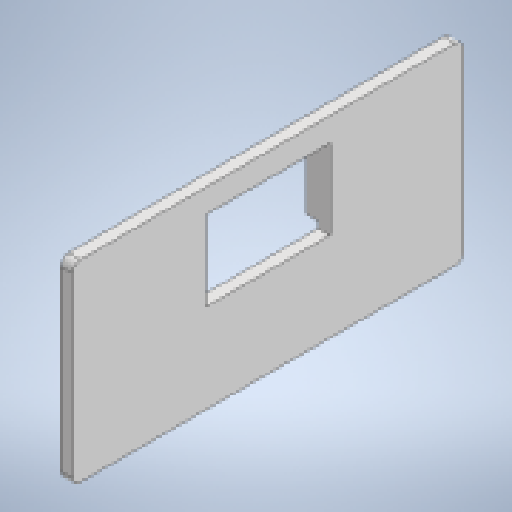
# Autodesk Inventor part: pokrywa_tyl
Saved by Autodesk Inventor 2023 (Build 270158000, 158)
## iProperties
Created: 2024-07-28
Part Number: pokrywa_tyl
Material: Ogólny
Document SubType Name: Modeling
Designer: kamil
Density: 1 g/cm^3
Appearance: Domyślna
Author: kamil
Autodesk Inventor part; units mm, degrees
ref_plane "YZ Plane" through (0, 0, 0) normal (1, 0, 0) x (0, 1, 0)
ref_plane "XZ Plane" through (0, 0, 0) normal (0, 1, 0) x (-1, 0, 0)
ref_plane "XY Plane" through (0, 0, 0) normal (0, 0, 1) x (1, 0, 0)
sketch "Szkic1" plane through (0, 0, 0) normal (1, 0, 0) x (0, 1, 0)
  line L0 (-29.4319, -23.6453) -> (19.8681, -23.6453)
  line L1 (19.8681, -23.6453) -> (19.8681, 76.3547)
  line L2 (19.8681, 76.3547) -> (-29.4319, 76.3547)
  line L3 (-29.4319, 76.3547) -> (-29.4319, -23.6453)
  point P0 (0, 0)
  dimension "d0" = 100
  dimension "d1" = 49.3
  constraints: 8 end point, 2 parallel, 1 horizontal, 1 perpendicular
  measures "d0" distance of L0.end L1.end
  measures "d1" distance between parallel lines of L3 L1
extrude "Wyciągnięcie proste1" add sketch "Szkic1" along normal blind 3
fillet "Zaokrąglenie1" radius 2 4 edges at (1.5, 19.8681, 76.3547) (1.5, -29.4319, 76.3547) (1.5, -29.4319, -23.6453) (1.5, 19.8681, -23.6453)
sketch "Szkic3" plane through (3, 0, 0) normal (1, 0, 0) x (0, 0, -1)
  line L0 (-10.6165, 13.5523) -> (-41.9165, 13.5523) projected
  line L1 (-41.9165, 13.5523) -> (-41.9165, -6.4477) projected
  line L2 (-41.9165, -6.4477) -> (-10.6165, -6.4477) projected
  line L3 (-10.6165, -6.4477) -> (-10.6165, 13.5523) projected
  line L4 (-42.1165, 13.7523) -> (-10.4165, 13.7523)
  line L5 (-10.4165, 13.7523) -> (-10.4165, -6.6477)
  line L6 (-10.4165, -6.6477) -> (-42.1165, -6.6477)
  line L7 (-42.1165, -6.6477) -> (-42.1165, 13.7523)
  point P0 (0, 0)
  dimension "d13" = 0.2
  constraints: 8 end point, 3 other
  measures "d13" distance between parallel lines of L0 L4
extrude "Wyciągnięcie proste2" cut sketch "Szkic3" against normal blind 3 contours L3 L2 L1 L0 | L4 L5 L6 L7
sketch "Szkic4" plane through (0, 0, 0) normal (-1, 0, 0) x (0, 0, 1)
  line L0 (5.5165, 12.0523) -> (5.5165, 6.0523) projected
  line L1 (5.5165, 6.0523) -> (4.5165, 6.0523) projected
  line L2 (4.5165, 6.0523) -> (4.5165, 1.0523) projected
  line L3 (4.5165, 1.0523) -> (5.5165, 1.0523) projected
  line L4 (5.5165, 1.0523) -> (5.5165, -4.9477) projected
  line L5 (5.5165, -4.9477) -> (47.0165, -4.9477) projected
  line L6 (47.0165, -4.9477) -> (47.0165, 1.0523) projected
  line L7 (47.0165, 1.0523) -> (48.0165, 1.0523) projected
  line L8 (48.0165, 1.0523) -> (48.0165, 6.0523) projected
  line L9 (48.0165, 6.0523) -> (47.0165, 6.0523) projected
  line L10 (47.0165, 6.0523) -> (47.0165, 12.0523) projected
  line L11 (47.0165, 12.0523) -> (5.5165, 12.0523) projected
  circle A0 centre (44.2665, 3.5523) radius 1.2 projected
  circle A1 centre (8.2665, 3.5523) radius 1.2 projected
  line L12 (10.4165, -6.6477) -> (10.4165, 13.7523) projected
  line L13 (10.4165, 13.7523) -> (42.1165, 13.7523) projected
  line L14 (42.1165, 13.7523) -> (42.1165, -6.6477) projected
  line L15 (42.1165, -6.6477) -> (10.4165, -6.6477) projected
  arc A2 (-21.6453, 19.8681) -> (-23.6453, 17.8681) centre (-21.6453, 17.8681) ccw projected
  line L16 (-23.6453, -27.4319) -> (-23.6453, 17.8681) projected
  arc A3 (-23.6453, -27.4319) -> (-21.6453, -29.4319) centre (-21.6453, -27.4319) ccw projected
  line L17 (74.3547, -29.4319) -> (-21.6453, -29.4319) projected
  arc A4 (74.3547, -29.4319) -> (76.3547, -27.4319) centre (74.3547, -27.4319) ccw projected
  line L18 (76.3547, 17.8681) -> (76.3547, -27.4319) projected
  arc A5 (76.3547, 17.8681) -> (74.3547, 19.8681) centre (74.3547, 17.8681) ccw projected
  line L19 (-21.6453, 19.8681) -> (74.3547, 19.8681) projected
  point P0 (0, 0)
  point P1 (42.1165, 12.0523)
  point P2 (42.1165, -4.9477)
  point P3 (10.4165, -4.9477)
  point P4 (10.4165, 12.0523)
ref_plane "Płaszczyzna konstrukcyjna1" through (-3, -4.9477, 4.5165) normal (1, 0, 0) x (0, 1, 0)
extrude "Wyciągnięcie proste3" add sketch "Szkic4" along normal up to surface (3 mm away) contours L11 L12 L5 L4 L3 L2 L1 L0 | L11 L10 L9 L8 L7 L6 L5 L14 | A0 | A1
sketch "Szkic5" plane through (-3, -4.9477, 10.4165) normal (-1, 0, 0) x (0, 0, 1)
  circle A0 centre (-2.15, 8.5) radius 1.2 projected
  circle A1 centre (33.85, 8.5) radius 1.2 projected
  point P0 (-10.4165, 4.9477)
hole "Otwór2" at (-3, 3.5523, 8.2665) at (-3, 3.5523, 44.2665) direction (1, 0, 0) diameter 1.3 depth 3 tip angle 118 countersink diameter 2 countersink angle 90
